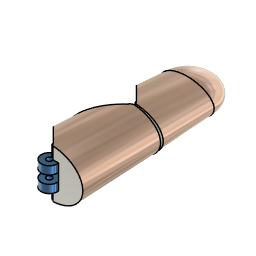
thumb assembly v1 (Autodesk Fusion 360 design; units mm, degrees)
Autodesk Fusion 360 part; units mm, degrees
sketch "base" plane through (0, 0, 0) normal (0, 1, 0) x (1, 0, 0) in component "thumb part 1 v2"
  ellipse E0 centre (0, 0) end of major axis (12, 0) minor radius 9
  line L0 (-12, 0) -> (12, 0) construction
  line L1 (0, -9) -> (0, 9) construction
  dimension "d1" = 24
  dimension "d2" = 18
  constraint coincident E0 L0.start
  constraint coincident E0 L0.end
  constraint coincident E0 L1.start
  constraint coincident E0 L1.end
  constraint coincident E0.centre origin
  constraint horizontal L0
  measures "d1" distance of E0
ref_plane "WorkPlane1" through (0, 30, 0) normal (0, 1, 0) x (1, 0, 0) in component "thumb part 1 v2"
sketch "top" plane through (0, 30, 0) normal (0, 1, 0) x (1, 0, 0) in component "thumb part 1 v2"
  ellipse E0 centre (0, 0) end of major axis (11, 0) minor radius 7.5
  line L0 (-11, 0) -> (11, 0) construction
  line L1 (0, -7.5) -> (0, 7.5) construction
  dimension "d4" = 22
  dimension "d5" = 15
  constraint coincident E0 L0.start
  constraint coincident E0 L0.end
  constraint coincident E0 L1.start
  constraint coincident E0 L1.end
  constraint coincident E0.centre origin
  constraint horizontal L0
  measures "d4" distance of E0
loft "Loft1" add profiles "top", "base" section 1 section 2 makes body 1 in component "thumb part 1 v2"
sketch "cut" plane through (0, 0, 0) normal (0, 0, 1) x (1, 0, 0) in component "thumb part 1 v2"
  line L0 (0, 30) -> (0, 30.5)
  line L1 (0, 0) -> (0, 1)
  line L2 (0, 1) -> (-14.1421, 15.1421)
  line L3 (0, 1) -> (20, 1) construction
  line L4 (-14.1421, 15.1421) -> (-14.1421, 0)
  line L5 (-14.1421, 0) -> (0, 0)
  line L6 (0, 0) -> (0, -0.5)
  line L7 (0, 30) -> (0, 29)
  line L8 (0, 29) -> (-14.1421, 14.8579)
  line L9 (0, 29) -> (20, 29) construction
  line L10 (0, 30) -> (-11.4565, 30)
  line L11 (-11.4565, 30) -> (-14.1421, 14.8579)
  dimension "d6" = 0.5
  dimension "d7" = 1
  dimension "d8" = 135
  dimension "d9" = 20
  dimension "d10" = 0.5
  dimension "d11" = 1
  dimension "d12" = 135
  dimension "d13" = 20
  constraint vertical L0
  constraint coincident L1.start L5.end
  constraint vertical L1
  constraint horizontal L3
  constraint parallel L1 L4
  constraint perpendicular L1 L5
  constraint perpendicular L5 L6
  constraint parallel L0 L7
  constraint horizontal L9
  constraint perpendicular L7 L10
  measures "d6" distance of L0.start L0.end
  measures "d7" distance of L1.start L1.end
  measures "d8" angle of L2 L3
  measures "d9" distance of L1.end L2.end
  measures "d10" distance of L1.start L6.end
  measures "d11" distance of L0.start L7.end
  measures "d12" angle of L8 L9
  measures "d13" distance of L7.end L8.end
extrude "Extrude1" cut sketch "cut" along normal mid plane 40 contours L1 L2 L4 L5 L8 | L2 L7 L8 L10 L11 bodies 1 in component "thumb part 1 v2"
sketch "wheel" plane through (0, 0, 0) normal (0, 0, 1) x (1, 0, 0) in component "thumb part 1 v2"
  line L0 (0, 0) -> (0, -0.5)
  circle A0 centre (0, -0.5) radius 3
  circle A1 centre (0.0423, 30.5794) radius 3
  dimension "d16" = 0.5
  dimension "d17" = 6
  dimension "d18" = 6
  constraint coincident L0.start origin
  constraint vertical L0
  constraint coincident L0.end A0.centre
  measures "d16" distance of L0.start L0.end
  measures "d17" diameter of A0
  measures "d18" diameter of A1
extrude "Extrude2" add sketch "wheel" along normal mid plane 3 separate body contours A1 makes body 2 in component "thumb part 1 v2"
extrude "Extrude3" cut sketch "wheel" along normal mid plane 3 contours A0 bodies 1 in component "thumb part 1 v2"
sketch "lower wheel offset" plane through (0, 0, -1.5) normal (0, 0, 1) x (-1, 0, 0) in component "thumb part 1 v2"
  line L0 (0, 0) -> (-2.958, 0)
  arc A0 (-2.958, 0) -> (1.2343, -2.2343) centre (0, 0.5) ccw
  line L1 (1.2343, -2.2343) -> (0, -1)
  line L2 (0, -1) -> (0, 0)
  circle A1 centre (0, 0.5) radius 3
  dimension "d23" = 6
  constraint concentric A0 A1
  measures "d23" diameter of A1
extrude "Extrude4" add sketch "lower wheel offset" against normal blind 3 separate body makes body 3 in component "thumb part 1 v2"
sketch "lower wheel offset2" plane through (0, 0, 1.5) normal (0, 0, -1) x (1, 0, 0) in component "thumb part 1 v2"
  line L0 (2.958, 0) -> (0, 0)
  line L1 (0, 0) -> (0, -1)
  line L2 (0, -1) -> (-1.2343, -2.2343)
  arc A0 (-1.2343, -2.2343) -> (2.958, 0) centre (0, 0.5) ccw
  circle A1 centre (0, 0.5) radius 3
  dimension "d26" = 6
  constraint concentric A0 A1
  measures "d26" diameter of A1
extrude "Extrude5" add sketch "lower wheel offset2" against normal blind 3 separate body makes body 4 in component "thumb part 1 v2"
sketch "rod cut" plane through (0, 0, 0) normal (0, 0, 1) x (1, 0, 0) in component "thumb part 1 v2"
  circle A0 centre (0, -0.5) radius 1
  circle A1 centre (0, 30.5) radius 1
  dimension "d29" = 2
  dimension "d30" = 2
  measures "d29" diameter of A0
  measures "d30" diameter of A1
extrude "Extrude6" cut sketch "rod cut" along normal mid plane 40 bodies 1 2 3 4 in component "thumb part 1 v2"
sketch "cut1" plane through (0, 0, 0) normal (0, 0, 1) x (1, 0, 0) in component "thumb part 1 v2"
  line L0 (-11.2352, 28.0792) -> (-12.0499, 0.073)
  line L1 (-11.2873, 26.2868) -> (-11.7871, 26.3013)
  line L2 (-11.7871, 26.3013) -> (-12.2837, 9.2286)
  line L3 (-12.2837, 9.2286) -> (-8.2854, 9.1123)
  line L4 (-8.2854, 9.1123) -> (-7.7373, 27.9536)
  line L5 (-7.7373, 27.9536) -> (-13.835, 22.4822)
  dimension "d34" = 0.5
  dimension "d35" = 4
  constraint coincident L0 L1.start
  constraint perpendicular L0 L1
  constraint perpendicular L1 L2
  constraint perpendicular L0 L3
  constraint perpendicular L3 L4
  measures "d34" distance of L1.start L1.end
  measures "d35" distance of L2.end L3.end
extrude "Extrude7" cut sketch "cut1" along normal mid plane 3 bodies 1 in component "thumb part 1 v2"
sketch "cut 2" plane through (0, 0, 0) normal (0, 0, 1) x (1, 0, 0) in component "thumb part 1 v2"
  line L0 (-10.8243, 28.0652) -> (-11.8243, 0.0652)
  line L1 (-11.0041, 23.0296) -> (-10.5045, 23.0118)
  line L2 (-10.5045, 23.0118) -> (-10.8675, 12.8473)
  line L3 (-10.8675, 12.8473) -> (-8.8688, 12.7759)
  line L4 (-8.8688, 12.7759) -> (-8.5885, 20.6232)
  line L5 (-8.5885, 20.6232) -> (-10.5045, 23.0118)
  dimension "d38" = 0.5
  dimension "d39" = 2
  constraint coincident L0 L1.start
  constraint perpendicular L0 L1
  constraint perpendicular L1 L2
  constraint perpendicular L2 L3
  constraint perpendicular L3 L4
  measures "d38" distance of L1.start L1.end
  measures "d39" distance of L2.end L3.end
extrude "Extrude8" cut sketch "cut 2" along normal mid plane 4 bodies 1 in component "thumb part 1 v2"
copy_body "Body->Comp1" bodies 1 removing the originals makes body 5 in component "index part 1"
copy_body "Body->Comp2" bodies 2 removing the originals makes body 6 in component "uppr wheel"
copy_body "Body->Comp3" bodies 3 removing the originals makes body 7 in component "lower wheel 1"
copy_body "Body->Comp4" bodies 4 removing the originals makes body 8 in component "lower wheel 2"
sketch "Sketch11" plane through (0, 0, 0) normal (0, 1, 0) x (1, 0, 0) in component "thumb part 1 v2"
extrude "Extrude1'" cut 1 faces at (0.7378, 32.769, 1.5) along direction (0, 0, 1) blind 3 on bodies 6 bodies 5 in component "index part 1"
extrude "Extrude2'" cut 1 faces at (0.7378, 32.769, -1.5) along direction (0, 0, -1) blind 3 on bodies 6 bodies 5 in component "index part 1"
combine "Combine1" operation add target body 5 tool bodies 8 7 6 in component "index part 1"
sketch "base (2)" plane through (0, 0, 0) normal (0, 1, 0) x (1, 0, 0) in component "thumb 2 v2"
  ellipse E0 centre (0, 0) end of major axis (11, 0) minor radius 7
  line L0 (-11, 0) -> (11, 0) construction
  line L1 (0, -7) -> (0, 7) construction
  dimension "d1_1" = 22
  dimension "d2_1" = 14
  constraint coincident E0 L0.start
  constraint coincident E0 L0.end
  constraint coincident E0 L1.start
  constraint coincident E0 L1.end
  constraint coincident E0.centre origin
  constraint horizontal L0
  measures "d1_1" distance of E0
ref_plane "WorkPlane1" through (0, 20, 0) normal (0, 1, 0) x (1, 0, 0) in component "thumb 2 v2"
sketch "top (2)" plane through (0, 20, 0) normal (0, 1, 0) x (1, 0, 0) in component "thumb 2 v2"
  ellipse E0 centre (0, 0) end of major axis (10, 0) minor radius 5.5
  line L0 (-10, 0) -> (10, 0) construction
  line L1 (0, -5.5) -> (0, 5.5) construction
  dimension "d4_1" = 20
  dimension "d5_1" = 11
  constraint coincident E0 L0.start
  constraint coincident E0 L0.end
  constraint coincident E0 L1.start
  constraint coincident E0 L1.end
  constraint coincident E0.centre origin
  constraint horizontal L0
  measures "d4_1" distance of E0
loft "Loft1'" add profiles "top (2)", "base (2)" section 1 section 2 separate body makes body 9 in component "thumb 2 v2"
sketch "cut (2)" plane through (0, 0, 0) normal (0, 0, 1) x (1, 0, 0) in component "thumb 2 v2"
  line L0 (0, 28) -> (0, 28.5)
  line L1 (0, 0) -> (0, 1)
  line L2 (0, 1) -> (-14.1421, 15.1421)
  line L3 (0, 1) -> (20, 1) construction
  line L4 (-14.1421, 15.1421) -> (-14.1421, 0)
  line L5 (-14.1421, 0) -> (0, 0)
  line L6 (0, 0) -> (0, -0.5)
  line L7 (0, 28) -> (0, 27)
  line L8 (0, 27) -> (20, 27) construction
  line L9 (0, 28) -> (-11.4565, 28)
  line L10 (-11.4565, 28) -> (-14.1421, 12.8579)
  dimension "d6_1" = 0.5
  dimension "d7_1" = 1
  dimension "d8_1" = 135
  dimension "d9_1" = 20
  dimension "d10_1" = 0.5
  dimension "d11_1" = 1
  dimension "d13_1" = 20
  constraint vertical L0
  constraint coincident L1.start L5.end
  constraint vertical L1
  constraint horizontal L3
  constraint parallel L1 L4
  constraint perpendicular L1 L5
  constraint perpendicular L5 L6
  constraint parallel L0 L7
  constraint horizontal L8
  constraint perpendicular L7 L9
  measures "d6_1" distance of L0.start L0.end
  measures "d7_1" distance of L1.start L1.end
  measures "d8_1" angle of L2 L3
  measures "d9_1" distance of L1.end L2.end
  measures "d10_1" distance of L1.start L6.end
  measures "d11_1" distance of L0.start L7.end
  measures "d13_1" distance of L7.end L10.end
extrude "Extrude1''" cut sketch "cut (2)" along normal mid plane 40 contours L1 L2 L4 L5 L10 bodies 9 in component "thumb 2 v2"
sketch "wheel (2)" plane through (0, 0, 0) normal (0, 0, 1) x (1, 0, 0) in component "thumb 2 v2"
  line L0 (0, 0) -> (0, -0.5)
  circle A0 centre (0, -0.5) radius 3
  dimension "d16_1" = 0.5
  dimension "d17_1" = 6
  constraint coincident L0.start origin
  constraint vertical L0
  constraint coincident L0.end A0.centre
  measures "d16_1" distance of L0.start L0.end
  measures "d17_1" diameter of A0
extrude "Extrude3'" cut sketch "wheel (2)" along normal mid plane 3 bodies 9 in component "thumb 2 v2"
sketch "lower wheel offset (2)" plane through (0, 0, -1.5) normal (0, 0, 1) x (-1, 0, 0) in component "thumb 2 v2"
  line L0 (0, 0) -> (-2.958, 0)
  arc A0 (-2.958, 0) -> (1.2343, -2.2343) centre (0, 0.5) ccw
  line L1 (0, -1) -> (0, 0)
  circle A1 centre (0, 0.5) radius 3
  line L2 (1.2343, -2.2343) -> (0, -1)
  dimension "d23_1" = 6
  constraint concentric A0 A1
  measures "d23_1" diameter of A1
extrude "Extrude4'" add sketch "lower wheel offset (2)" against normal blind 3 separate body makes body 10 in component "thumb 2 v2"
sketch "lower wheel offset2 (2)" plane through (0, 0, 1.5) normal (0, 0, -1) x (1, 0, 0) in component "thumb 2 v2"
  line L0 (2.958, 0) -> (0, 0)
  line L1 (0, 0) -> (0, -1)
  arc A0 (-1.2343, -2.2343) -> (2.958, 0) centre (0, 0.5) ccw
  circle A1 centre (0, 0.5) radius 3
  line L2 (0, -1) -> (-1.2343, -2.2343)
  dimension "d26_1" = 6
  constraint concentric A0 A1
  measures "d26_1" diameter of A1
extrude "Extrude5'" add sketch "lower wheel offset2 (2)" against normal blind 3 separate body makes body 11 in component "thumb 2 v2"
sketch "rod cut (2)" plane through (0, 0, 0) normal (0, 0, 1) x (1, 0, 0) in component "thumb 2 v2"
  circle A0 centre (0, -0.5) radius 1
  dimension "d29_1" = 2
  measures "d29_1" diameter of A0
copy_body "Body->Comp1'" bodies 9 removing the originals makes body 12 in component "index part 1 (1)"
copy_body "Body->Comp3'" bodies 10 removing the originals makes body 13 in component "lower wheel 1 (1)"
copy_body "Body->Comp4'" bodies 11 removing the originals makes body 14 in component "lower wheel 2 (1)"
sketch "Sketch12" plane through (0, 20, 0) normal (0, 1, 0) x (-1, 0, 0) in component "thumb 2 v2"
  ellipse E0 centre (0, 0) end of major axis (-10, 0) minor radius 5.5
  line L0 (0, -5.5) -> (0, 5.5)
  ellipse E1 centre (0, 0) end of major axis (-10, 0) minor radius 5.5 (0, 5.5) -> (0, -5.5) ccw
  dimension "d46" = 20
  dimension "d47" = 11
  constraint coincident E0.centre E1.centre
  measures "d46" distance of E1
revolve "Revolve1" add sketch "Sketch12" angle 180 about axis through (0, 20, -5.5) along (0, 0, 1) contours E0 L0 E1 bodies 12 in component "index part 1 (1)"
extrude "Extrude3''" cut sketch "rod cut (2)" along normal mid plane 40 bodies 12 in component "index part 1 (1)"
extrude "Extrude1'''" cut sketch "rod cut (2)" along normal mid plane 40 bodies 13 in component "lower wheel 1 (1)"
extrude "Extrude1''''" cut sketch "rod cut (2)" along normal mid plane 40 bodies 14 in component "lower wheel 2 (1)"
combine "Combine1'" operation add target body 12 tool bodies 13 14 in component "index part 1 (1)"
component "thumb part 1 v2" placed x (1, 0, 0) y (0, 1, 0) z (0, 0, 1) at (0, 0, 0)
component "thumb 2 v2" placed x (1, 0, 0) y (0, 1, 0) z (0, 0, 1) at (0, 0, 0)
component "index part 1" placed x (1, 0, 0) y (0, 1, 0) z (0, 0, 1) at (12.7576, 5.5566, -7.201) in component "thumb part 1 v2"
component "uppr wheel" placed x (1, 0, 0) y (0, 1, 0) z (0, 0, 1) at (0, 0, 0) in component "thumb part 1 v2"
component "lower wheel 1" placed x (1, 0, 0) y (0, 1, 0) z (0, 0, 1) at (0, 0, 0) in component "thumb part 1 v2"
component "lower wheel 2" placed x (1, 0, 0) y (0, 1, 0) z (0, 0, 1) at (0, 0, 0) in component "thumb part 1 v2"
component "index part 1 (1)" placed x (1, 0, 0) y (0, 1, 0) z (0, 0, 1) at (12.7576, 36.5566, -7.201) in component "thumb 2 v2"
component "lower wheel 1 (1)" placed x (1, 0, 0) y (0, 1, 0) z (0, 0, 1) at (0, 0, 0) in component "thumb 2 v2"
component "lower wheel 2 (1)" placed x (1, 0, 0) y (0, 1, 0) z (0, 0, 1) at (0, 0, 0) in component "thumb 2 v2"
named bodies: "index part 1", "uppr wheel", "lower wheel 1", "lower wheel 2"
